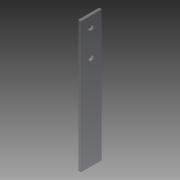
# Autodesk Inventor part: Polycarbonate Battery Spacer
Saved by Autodesk Inventor 2013 (Build 170138000, 138)
## iProperties
Created: 2013-02-09
Part Number: Polycarbonate Battery Spacer
Material: Polycarbonate, Clear
Document SubType Name: Modeling
Designer: Moses
Mass: 11.2509 g
Surface Area: 92.2858 cm^2
Volume: 12.5849 cm^3
Density: 0.894 g/cm^3
Author: Moses
Autodesk Inventor part; units mm, degrees
ref_plane "YZ Plane" through (0, 0, 0) normal (1, 0, 0) x (0, 1, 0)
ref_plane "XZ Plane" through (0, 0, 0) normal (0, 1, 0) x (-1, 0, 0)
ref_plane "XY Plane" through (0, 0, 0) normal (0, 0, 1) x (1, 0, 0)
sketch "Sketch1" plane through (0, 0, 0) normal (1, 0, 0) x (0, 1, 0)
  line L0 (0, 0) -> (158.75, 0)
  line L1 (158.75, 0) -> (158.75, 25.4)
  line L2 (158.75, 25.4) -> (0, 25.4)
  line L3 (0, 25.4) -> (0, 0)
  line L4 (0, 12.7) -> (158.75, 12.7) construction
  circle A0 centre (146.05, 12.7) radius 3.302
  circle A1 centre (114.3, 12.7) radius 3.302
  dimension "d0" = 158.75
  dimension "d2" = 25.4
  dimension "d3" = 6.604
  dimension "d4" = 12.7
  dimension "d5" = 31.75
  constraints: 10 end point, 2 centre point, 2 midpoint, 2 parallel, 2 point on line, 1 equal radius, 1 horizontal, 1 perpendicular
  measures "d0" distance of L1.end L2.end
  measures "d2" distance of L2.end L0.start
  measures "d3" diameter of A0
  measures "d4" distance from line of L1 A0.centre
  measures "d5" distance of A0.centre A1.centre
extrude "Extrusion1" add sketch "Sketch1" along normal blind 3.175
body "Solid1"
